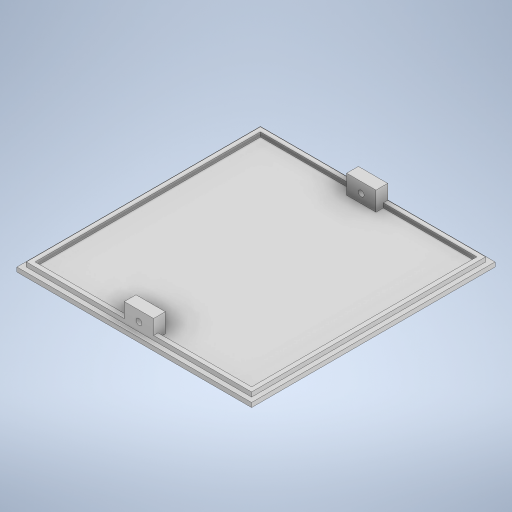
# Autodesk Inventor part: Gyrosensor_Deckel
Saved by Autodesk Inventor 2024 (Build 280153000, 153)
## iProperties
Created: 2024-03-07
Part Number: Gyrosensor_Deckel
Material: Generisch
Document SubType Name: Modeling
Designer: User
Density: 1 g/cm^3
Appearance: Vorgabe
Author: User
Autodesk Inventor part; units mm, degrees
ref_plane "YZ Plane" through (0, 0, 0) normal (1, 0, 0) x (0, 1, 0)
ref_plane "XZ Plane" through (0, 0, 0) normal (0, 1, 0) x (-1, 0, 0)
ref_plane "XY Plane" through (0, 0, 0) normal (0, 0, 1) x (1, 0, 0)
sketch "Skizze1" plane through (0, 0, 0) normal (0, 0, 1) x (1, 0, 0)
  line L0 (-40.0777, 35.7212) -> (39.9223, 35.7212)
  line L1 (39.9223, 35.7212) -> (39.9223, -47.2788)
  line L2 (39.9223, -47.2788) -> (-40.0777, -47.2788)
  line L3 (-40.0777, -47.2788) -> (-40.0777, 35.7212)
  line L4 (-38.4777, 34.1212) -> (38.3223, 34.1212)
  line L5 (38.3223, 34.1212) -> (38.3223, -45.6788)
  line L6 (38.3223, -45.6788) -> (-38.4777, -45.6788)
  line L7 (-38.4777, -45.6788) -> (-38.4777, 34.1212)
  line L8 (-36.9777, 32.6212) -> (36.8223, 32.6212)
  line L9 (36.8223, 32.6212) -> (36.8223, -44.1788)
  line L10 (36.8223, -44.1788) -> (-36.9777, -44.1788)
  line L11 (-36.9777, -44.1788) -> (-36.9777, 32.6212)
  line L12 (-5.0777, -45.6788) -> (4.9223, -45.6788)
  line L13 (4.9223, -45.6788) -> (4.9223, -41.6788)
  line L14 (4.9223, -41.6788) -> (-5.0777, -41.6788)
  line L15 (-5.0777, -41.6788) -> (-5.0777, -45.6788)
  line L16 (-5.0777, 34.1212) -> (4.9223, 34.1212)
  line L17 (4.9223, 34.1212) -> (4.9223, 30.1212)
  line L18 (4.9223, 30.1212) -> (-5.0777, 30.1212)
  line L19 (-5.0777, 30.1212) -> (-5.0777, 34.1212)
  point P0 (0, 0)
  point P1 (-0.0777, -41.6788)
  point P2 (-0.0777, 30.1212)
  point P3 (4.9223, 32.6212)
  point P4 (-5.0777, 32.6212)
  point P5 (-5.0777, -44.1788)
  point P6 (4.9223, -44.1788)
  dimension "d0" = 80
  dimension "d1" = 83
  dimension "d2" = 1.6
  dimension "d3" = 1.5
  dimension "d4" = 1.6
  dimension "d5" = 1.5
  dimension "d6" = 1.6
  dimension "d7" = 1.5
  dimension "d8" = 1.6
  dimension "d9" = 1.5
  dimension "d10" = 10
  dimension "d11" = 4
  dimension "d12" = 40
  dimension "d13" = 4
  dimension "d14" = 10
  dimension "d16" = 40
  constraints: 40 end point, 10 parallel, 5 horizontal, 5 perpendicular, 2 midpoint, 2 point on line
  measures "d0" distance of L0.start L0.end
  measures "d1" distance of L0.end L1.end
  measures "d2" distance between parallel lines of L0 L4
  measures "d3" distance between parallel lines of L4 L8
  measures "d4" distance between parallel lines of L1 L5
  measures "d5" distance between parallel lines of L5 L9
  measures "d6" distance between parallel lines of L3 L7
  measures "d7" distance between parallel lines of L11 L7
  measures "d8" distance between parallel lines of L2 L6
  measures "d9" distance between parallel lines of L6 L10
  measures "d10" distance of L13.end L14.end
  measures "d11" distance of L12.end L13.end
  measures "d12" distance from line of L1 point (-0.078, -41.679)
  measures "d13" distance of L16.end L17.end
  measures "d14" distance of L17.end L18.end
  measures "d16" distance from line of L1 point (-0.078, 30.121)
extrude "Extrusion1" add sketch "Skizze1" along normal blind 1.5 contours L0 L1 L2 L3 | L19 L18 L17 L8 L9 L10 L13 L14 L15 L11
extrude "Extrusion2" add sketch "Skizze1" along normal blind 3 contours L4 L19 L8 L11 L10 L15 L6 L7 | L4 L5 L6 L13 L10 L9 L8 L17
extrude "Extrusion3" add sketch "Skizze1" along normal blind 8 contours L4 L17 L8 L19 | L8 L17 L18 L19 | L15 L10 L13 L6 | L15 L14 L13 L10
sketch "Skizze2" plane through (-38.4777, -45.6788, 1.5) normal (0, -1, 0) x (1, 0, 0)
  circle A0 centre (38.4, 3) radius 1
  line L0 (-1.6, 0) -> (78.4, 0) projected
  line L1 (33.4, 1.5) -> (33.4, 6.5) projected
  point P0 (38.4777, -1.5)
  dimension "d23" = 2
  dimension "d24" = 3
  dimension "d25" = 5
  constraints: 1 centre point
  measures "d23" diameter of A0
  measures "d24" distance from line of A0.centre L0
  measures "d25" distance from line of L1 A0.centre
extrude "Extrusion4" cut sketch "Skizze2" against normal through all
